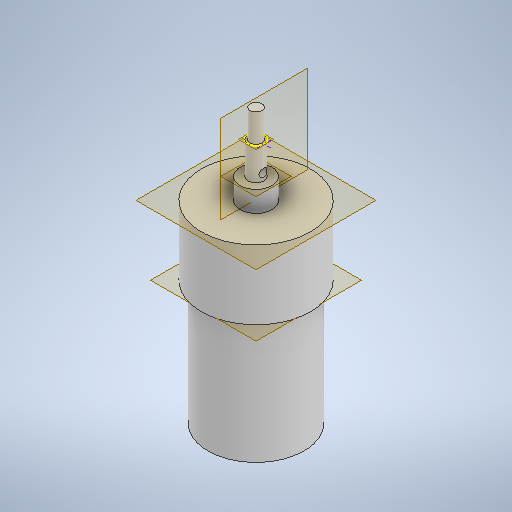
# Autodesk Inventor part: daisen_motor
Saved by Autodesk Inventor 2025.2 (Build 292293000, 293)
## iProperties
Created: 2024-12-21
Part Number: daisen_motor
Material: 一般
Document SubType Name: Modeling
Designer: mahhy
Density: 1 g/cm^3
Appearance: 既定
Author: mahhy
Autodesk Inventor part; units mm, degrees
ref_plane "YZ Plane" through (0, 0, 0) normal (1, 0, 0) x (0, 1, 0)
ref_plane "XZ Plane" through (0, 0, 0) normal (0, 1, 0) x (-1, 0, 0)
ref_plane "XY Plane" through (0, 0, 0) normal (0, 0, 1) x (1, 0, 0)
sketch "スケッチ8" plane through (0, 0, 0) normal (0, 1, 0) x (-1, 0, 0)
  circle A0 centre (0, 0) radius 12
  dimension "d29" = 24
  constraints: 1 centre point, 1 coincident
  measures "d29" diameter of A0
extrude "押し出し6" add sketch "スケッチ8" along normal blind 31
ref_plane "作業平面4" through (0, 31, 0) normal (0, 1, 0) x (1, 0, 0)
sketch "スケッチ9" plane through (0, 31, 0) normal (0, 1, 0) x (1, 0, 0)
  circle A0 centre (0, 0) radius 13.65
  dimension "d33" = 27.3
  constraints: 1 centre point, 1 coincident
  measures "d33" diameter of A0
extrude "押し出し7" add sketch "スケッチ9" along normal blind 17.3
ref_plane "作業平面5" through (0, 48.3, 0) normal (0, 1, 0) x (1, 0, 0)
sketch "スケッチ10" plane through (0, 48.3, 0) normal (0, 1, 0) x (1, 0, 0)
  circle A0 centre (0, 0) radius 4
  dimension "d37" = 8
  constraints: 1 centre point, 1 coincident
  measures "d37" diameter of A0
extrude "押し出し8" add sketch "スケッチ10" along normal blind 5.2
ref_plane "作業平面6" through (0, 53.5, 0) normal (0, 1, 0) x (1, 0, 0)
sketch "スケッチ11" plane through (0, 53.5, 0) normal (0, 1, 0) x (1, 0, 0)
  circle A0 centre (0, 0) radius 2
  dimension "d41" = 4
  constraints: 1 centre point, 1 coincident
  measures "d41" diameter of A0
extrude "押し出し9" add sketch "スケッチ11" along normal blind 8
ref_plane "作業平面7" through (0, 61.5, 0) normal (0, 1, 0) x (1, 0, 0)
sketch "スケッチ12" plane through (0, 61.5, 0) normal (0, 1, 0) x (1, 0, 0)
  circle A0 centre (0, 0) radius 1.5
  dimension "d45" = 3
  constraints: 1 centre point, 1 coincident
  measures "d45" diameter of A0
extrude "押し出し10" add sketch "スケッチ12" along normal blind 7
sketch "スケッチ13" plane through (0, 61.5, 0) normal (0, 1, 0) x (1, 0, 0)
  circle A0 centre (0, 0) radius 2 projected
  point P0 (2, 0)
  constraints: 1 horizontal alignment, 1 other
ref_plane "作業平面8" through (2, 61.5, 0) normal (1, 0, 0) x (0, 1, 0)
sketch "スケッチ14" plane through (2, 61.5, 0) normal (1, 0, 0) x (0, 1, 0)
  circle A0 centre (-6.2, 0) radius 1
  line L0 (0, -2) -> (0, 2) projected
  point P0 (-61.5, 0)
  dimension "d48" = 2
  dimension "d49" = 6.2
  constraints: 1 centre point
  measures "d48" diameter of A0
  measures "d49" distance from line of A0.centre L0
hole "穴2" at (2, 55.3, 0) direction (-1, 0, 0) diameter 2 end through all
